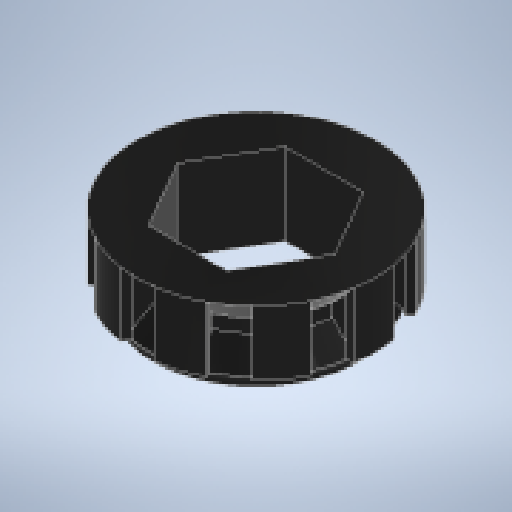
# Autodesk Inventor part: Tire Hub
Saved by Autodesk Inventor 2023.2 (Build 272271000, 271)
## iProperties
Created: 2023-02-06
Part Number: Tire Hub
Material: Nylon 6/6
Document SubType Name: Modeling
Designer: Nathan Cai
Density: 1.13 g/cm^3
Appearance: Smooth - Black
Mass: 3.14977 g
Surface Area: 28.8521 cm^2
Volume: 2.7874 cm^3
Wheel_OD: 1.000 in
Author: Nathan Cai
Autodesk Inventor part; units mm, degrees
ref_plane "YZ Plane" through (0, 0, 0) normal (1, 0, 0) x (0, 1, 0)
ref_plane "XZ Plane" through (0, 0, 0) normal (0, 1, 0) x (-1, 0, 0)
ref_plane "XY Plane" through (0, 0, 0) normal (0, 0, 1) x (1, 0, 0)
sketch "Sketch10" plane through (0, 0, 0) normal (0, 1, 0) x (-1, 0, 0)
  circle A0 centre (0, 0) radius 12.7 construction
  line L0 (0, 0) -> (12.7, 0) construction
  line L1 (7.3323, 0) -> (3.6662, -6.35)
  line L2 (3.6662, -6.35) -> (-3.6662, -6.35)
  line L3 (-3.6662, -6.35) -> (-7.3323, 0)
  line L4 (-7.3323, 0) -> (-3.6662, 6.35)
  line L5 (-3.6662, 6.35) -> (3.6662, 6.35)
  line L6 (3.6662, 6.35) -> (7.3323, 0)
  circle A1 centre (0, 0) radius 7.9375
  arc A2 (10.9437, -1.9297) -> (10.9437, 1.9297) centre (0, 0) ccw
  arc A3 (10.162, -1.7918) -> (10.162, 1.7918) centre (0, 0) ccw
  line L7 (7.8977, 0.7937) -> (10.2882, 0.7938)
  line L8 (11.0841, 9.7511) -> (11.0841, -0.7937) construction
  line L9 (10.2882, -0.7938) -> (7.8977, -0.7937)
  line L10 (10.162, 1.7918) -> (10.9437, 1.9297)
  line L11 (10.162, -1.7918) -> (10.9437, -1.9297)
  line L12 (5.9228, 5.2843) -> (7.8568, 6.6894)
  line L13 (8.7899, 5.4051) -> (6.8559, 4)
  line L14 (7.168, 7.4227) -> (7.7194, 7.9937)
  arc A4 (9.2744, 4.5234) -> (7.168, 7.4227) centre (0, 0) ccw
  line L15 (3.2357, 14.4039) -> (9.4338, 5.8729) construction
  line L16 (9.2744, 4.5234) -> (9.9878, 4.8714)
  arc A5 (9.9878, 4.8714) -> (7.7194, 7.9937) centre (0, 0) ccw
  line L17 (1.6856, 7.7565) -> (2.4243, 10.0299)
  line L18 (3.9341, 9.5394) -> (3.1954, 7.2659)
  line L19 (1.4361, 10.2183) -> (1.5466, 11.0044)
  arc A6 (4.8444, 9.1109) -> (1.4361, 10.2183) centre (0, 0) ccw
  line L20 (-5.8486, 13.5549) -> (4.1801, 10.2963) construction
  line L21 (4.8444, 9.1109) -> (5.217, 9.8118)
  arc A7 (5.217, 9.8118) -> (1.5466, 11.0044) centre (0, 0) ccw
  line L22 (-3.1954, 7.2659) -> (-3.9341, 9.5394)
  line L23 (-2.4243, 10.0299) -> (-1.6856, 7.7565)
  line L24 (-4.8444, 9.1109) -> (-5.217, 9.8118)
  arc A8 (-1.4361, 10.2183) -> (-4.8444, 9.1109) centre (0, 0) ccw
  line L25 (-12.699, 7.5284) -> (-2.6703, 10.7869) construction
  line L26 (-1.4361, 10.2183) -> (-1.5466, 11.0044)
  arc A9 (-1.5466, 11.0044) -> (-5.217, 9.8118) centre (0, 0) ccw
  line L27 (-6.8559, 4) -> (-8.7899, 5.4051)
  line L28 (-7.8568, 6.6894) -> (-5.9228, 5.2843)
  line L29 (-9.2744, 4.5234) -> (-9.9878, 4.8714)
  arc A10 (-7.168, 7.4227) -> (-9.2744, 4.5234) centre (0, 0) ccw
  line L30 (-14.6988, -1.3737) -> (-8.5007, 7.1572) construction
  line L31 (-7.168, 7.4227) -> (-7.7194, 7.9937)
  arc A11 (-7.7194, 7.9937) -> (-9.9878, 4.8714) centre (0, 0) ccw
  line L32 (-7.8977, -0.7938) -> (-10.2882, -0.7937)
  line L33 (-10.2882, 0.7937) -> (-7.8977, 0.7937)
  line L34 (-10.162, -1.7918) -> (-10.9437, -1.9297)
  arc A12 (-10.162, 1.7918) -> (-10.162, -1.7918) centre (0, 0) ccw
  line L35 (-11.0841, -9.7511) -> (-11.0841, 0.7937) construction
  line L36 (-10.162, 1.7918) -> (-10.9437, 1.9297)
  arc A13 (-10.9437, 1.9297) -> (-10.9437, -1.9297) centre (0, 0) ccw
  line L37 (-5.9228, -5.2843) -> (-7.8568, -6.6894)
  line L38 (-8.7899, -5.4051) -> (-6.8559, -4)
  line L39 (-7.168, -7.4227) -> (-7.7194, -7.9937)
  arc A14 (-9.2744, -4.5234) -> (-7.168, -7.4227) centre (0, 0) ccw
  line L40 (-3.2357, -14.4039) -> (-9.4338, -5.8729) construction
  line L41 (-9.2744, -4.5234) -> (-9.9878, -4.8714)
  arc A15 (-9.9878, -4.8714) -> (-7.7194, -7.9937) centre (0, 0) ccw
  line L42 (-1.6856, -7.7565) -> (-2.4243, -10.0299)
  line L43 (-3.9341, -9.5394) -> (-3.1954, -7.2659)
  line L44 (-1.4361, -10.2183) -> (-1.5466, -11.0044)
  arc A16 (-4.8444, -9.1109) -> (-1.4361, -10.2183) centre (0, 0) ccw
  line L45 (5.8486, -13.5549) -> (-4.1801, -10.2963) construction
  line L46 (-4.8444, -9.1109) -> (-5.217, -9.8118)
  arc A17 (-5.217, -9.8118) -> (-1.5466, -11.0044) centre (0, 0) ccw
  line L47 (3.1954, -7.2659) -> (3.9341, -9.5394)
  line L48 (2.4243, -10.0299) -> (1.6856, -7.7565)
  line L49 (4.8444, -9.1109) -> (5.217, -9.8118)
  arc A18 (1.4361, -10.2183) -> (4.8444, -9.1109) centre (0, 0) ccw
  line L50 (12.699, -7.5284) -> (2.6703, -10.7869) construction
  line L51 (1.4361, -10.2183) -> (1.5466, -11.0044)
  arc A19 (1.5466, -11.0044) -> (5.217, -9.8118) centre (0, 0) ccw
  line L52 (6.8559, -4) -> (8.7899, -5.4051)
  line L53 (7.8568, -6.6894) -> (5.9228, -5.2843)
  line L54 (9.2744, -4.5234) -> (9.9878, -4.8714)
  arc A20 (7.168, -7.4227) -> (9.2744, -4.5234) centre (0, 0) ccw
  line L55 (14.6988, 1.3737) -> (8.5007, -7.1572) construction
  line L56 (7.168, -7.4227) -> (7.7194, -7.9937)
  arc A21 (7.7194, -7.9937) -> (9.9878, -4.8714) centre (0, 0) ccw
  point P0 (6.8559, -4)
  point P1 (3.1954, 7.2659)
  point P2 (-1.6856, 7.7565)
  point P3 (-3.1954, 7.2659)
  point P4 (-5.9228, 5.2843)
  point P5 (-6.8559, 4)
  point P6 (-7.8977, 0.7937)
  point P7 (-7.8977, -0.7938)
  point P8 (-6.8559, -4)
  point P9 (-5.9228, -5.2843)
  point P10 (-3.1954, -7.2659)
  point P11 (-1.6856, -7.7565)
  point P12 (1.6856, -7.7565)
  point P13 (3.1954, -7.2659)
  dimension "Wheel_OD" = 25.4
  dimension "d65" = 12.7
  dimension "d66" = 15.875
  dimension "d67" = 22.225
  dimension "d68" = 0.7937
  dimension "d69" = 1.5875
  dimension "d71" = 10
  dimension "d74" = 360
  constraints: 114 end point, 72 point on circle, 21 centre point, 21 point on line, 15 coincident, 2 horizontal, 1 horizontal alignment, 1 parallel, 1 perpendicular, 216 other
  measures "d65" distance between parallel lines of L5 L2
  measures "d66" diameter of A1
  measures "d67" diameter of A2
  measures "d68" radial gap between concentric circles of A2 A3
  measures "d69" distance between parallel lines of L7 L9
  measures "d71" angle of L9 L11
extrude "Extrusion7" add sketch "Sketch10" along normal blind 7.62 contours A1
sketch "Sketch11" plane through (0, 7.62, 0) normal (0, 1, 0) x (1, 0, 0)
  circle A0 centre (0, 0) radius 11.1125
  circle A1 centre (0, 0) radius 7.9375
  dimension "d78" = 22.225
  dimension "d79" = 15.875
  constraints: 2 centre point, 2 coincident
  measures "d78" diameter of A0
  measures "d79" diameter of A1
extrude "Extrusion8" add sketch "Sketch11" against normal blind 3.175
chamfer "Chamfer5" distance 3.175 angle 45 1 edges at (-11.1125, 4.445, 0)
ref_plane "Work Plane4" through (0, 3.81, 0) normal (0, -1, 0) x (1, 0, 0)
mirror "Mirror2" about plane through (0, 3.81, 0) normal (0, -1, 0) of "Extrusion8", "Chamfer5"
extrude "Extrusion9" add sketch "Sketch10" along normal up to surface (7.62 mm away) contours A1 L7 A3 L9 | A1 L12 A4 L13 | A3 L10 A2 L11 | L52 A20 L53 A1 | A4 L14 A5 L16 | A20 L54 A21 L56 | A1 L17 A6 L18 | L47 A18 L48 A1 | A6 L19 A7 L21 | A18 L49 A19 L51 | A1 L22 A8 L23 | L42 A16 L43 A1 | A8 L24 A9 L26 | A16 L44 A17 L46 | A1 L27 A10 L28 | L37 A14 L38 A1 | A10 L29 A11 L31 | A14 L39 A15 L41 | A1 L32 A12 L33 | A12 L34 A13 L36
sketch "Sketch13" plane through (0, 0, 0) normal (1, 0, 0) x (0, 1, 0)
  line L0 (0, 0) -> (0, 6.35) projected
  line L1 (0, -11.0044) -> (0, -9.8118) projected
  line L2 (0, 0) -> (0, -11.0044)
  line L3 (0, -6.35) -> (0, 0) projected
  circle A0 centre (0, -11.1125) radius 1.5875
  line L4 (0, -1.9297) -> (0, 1.9297) projected
  line L5 (0, 0) -> (-10.6988, 0) construction
  dimension "d91" = 3.175
  dimension "d92" = 11.1125
  constraints: 4 end point, 1 centre point, 1 horizontal, 1 midpoint, 1 point on line, 1 vertical
  measures "d91" diameter of A0
  measures "d92" distance of L5.start A0.centre
revolve "Revolution2" cut sketch "Sketch13" angle 360 about axis through (0, 0, 0) along (0, -1, 0)
body "Solid2"
